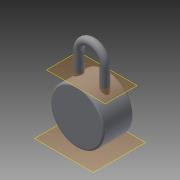
# Autodesk Inventor part: Noke
Saved by Autodesk Inventor 2015 SP2 (Build 190223200, 223)
## iProperties
Created: 2016-08-30
Part Number: Noke
Material: Generic
Document SubType Name: Modeling
Designer: jm799
Density: 1 g/cm^3
Appearance: Default
Author: jm799
Autodesk Inventor part; units mm, degrees
ref_plane "YZ Plane" through (0, 0, 0) normal (1, 0, 0) x (0, 1, 0)
ref_plane "XZ Plane" through (0, 0, 0) normal (0, 1, 0) x (-1, 0, 0)
sketch "Sketch1" plane through (0, 0, 0) normal (0, 1, 0) x (-1, 0, 0)
  circle A0 centre (0, 0) radius 27.375
  dimension "d0" = 54.75
  constraints: 1 centre point, 1 coincident
  measures "d0" diameter of A0
extrude "Extrusion1" add sketch "Sketch1" along normal blind 29.57
sketch "Sketch2" plane through (0, 29.57, 0) normal (0, 1, 0) x (1, 0, 0)
  point P0 (0, 0)
ref_plane "Work Plane1" through (0, 0, 27.375) normal (0, 0, 1) x (1, 0, 0)
sketch "Sketch3" plane through (0, 0, 27.375) normal (0, 0, 1) x (1, 0, 0)
  line L0 (-27.375, 0) -> (27.375, 0) construction
  line L1 (27.375, 0) -> (27.375, 29.57) construction
  line L2 (27.375, 0) -> (27.375, 29.57) construction
  line L3 (27.375, 29.57) -> (-27.375, 29.57) construction
  line L4 (-17.35, 14.785) -> (17.35, 14.785)
  circle A0 centre (13.3672, 14.785) radius 4
  line L5 (0, 0) -> (0, 29.57) construction
  circle A1 centre (-13.3672, 14.785) radius 4
  point P0 (0, 0)
  point P1 (0, 14.785)
  dimension "d3" = 34.7
  dimension "d4" = 8
  constraints: 7 end point, 3 midpoint, 2 centre point, 2 point on line, 1 horizontal, 1 perpendicular, 1 symmetric about line, 1 vertical alignment, 1 other
  measures "d3" distance of L4.start L4.end
  measures "d4" diameter of A0
extrude "Extrusion2" add sketch "Sketch3" against normal blind 10 and the other way blind 18
sketch "Sketch4" plane through (13.3672, 14.785, 45.375) normal (0, 0, 1) x (1, 0, 0)
  line L0 (-13.3672, -26.0897) -> (-13.3672, 22.3589)
  point P0 (-13.3672, -14.785)
  constraints: 2 end point, 1 vertical
sketch "Sketch5" plane through (13.3672, 14.785, 45.375) normal (0, 0, 1) x (1, 0, 0)
  circle A0 centre (0, 0) radius 4
  line L0 (-13.3672, 32.0486) -> (-13.3672, -35.7794) projected
  point P0 (-13.3672, -14.785)
  dimension "d9" = 8
  constraints: 1 centre point
  measures "d9" diameter of A0
revolve "Revolution1" add sketch "Sketch5" angle 180 about axis through (0, 37.1439, 45.375) along (0, -1, 0)
sketch "Sketch8" plane through (0, 0, 0) normal (0, -1, 0) x (1, 0, 0)
  circle A0 centre (0, 0) radius 26.75
  dimension "d11" = 53.5
  constraints: 1 centre point, 1 coincident
  measures "d11" diameter of A0
sketch "Sketch9" plane through (0, 29.57, 0) normal (0, 1, 0) x (1, 0, 0)
  circle A0 centre (0, 0) radius 26.75
  dimension "d12" = 53.5
  constraints: 1 centre point, 1 coincident
  measures "d12" diameter of A0
extrude "Extrusion3" add sketch "Sketch9" along normal blind 0.5
extrude "Extrusion4" add sketch "Sketch8" along normal blind 0.5
fillet "Fillet1" radius 2 1 edges at (-26.75, -0.5, 0)
fillet "Fillet2" radius 1.5 1 edges at (27.375, 0, 0)
fillet "Fillet3" radius 1.5 1 edges at (27.375, 29.57, 0)
fillet "Fillet4" radius 1 1 edges at (-26.75, 30.07, 0)
ref_plane "Work Plane2" through (0, 0, -27.375) normal (0, 0, 1) x (1, 0, 0)
sketch "Sketch10" plane through (0, 0, -27.375) normal (0, 0, 1) x (1, 0, 0)
  line L0 (27.375, 28.3517) -> (-27.375, 28.3517) construction
  line L1 (27.3423, 28.3517) -> (-27.3423, 28.3517) construction
  line L2 (27.375, 28.3517) -> (27.375, 1.2183) construction
  line L3 (-27.375, 1.2183) -> (27.375, 1.2183) construction
  line L4 (27.375, 1.2183) -> (27.375, 28.3517) construction
  circle A0 centre (0, 14.785) radius 7.5
  circle A1 centre (0, 14.785) radius 6.5
  line L5 (1.0367, 18.8545) -> (1.0367, 10.785)
  line L6 (-13.3672, 10.785) -> (13.3672, 10.785) projected
  line L7 (0, 28.3517) -> (0, 1.2183) construction
  line L8 (-1.0367, 18.8545) -> (-1.0367, 10.785)
  arc A2 (1.0367, 18.8545) -> (-1.0367, 18.8545) centre (0, 18.8545) ccw construction
  arc A3 (-1.0367, 10.785) -> (1.0367, 10.785) centre (0, 10.785) ccw construction
  arc A4 (1.0367, 18.8545) -> (-1.0367, 18.8545) centre (0, 18.8545) ccw
  arc A5 (-1.0367, 10.785) -> (1.0367, 10.785) centre (0, 10.785) ccw
  point P0 (0, 0)
  point P1 (0, 14.785)
  point P2 (27.375, 14.785)
  dimension "d21" = 15
  dimension "d22" = 13
  constraints: 11 end point, 8 point on circle, 6 centre point, 6 tangent, 4 midpoint, 3 point on line, 2 symmetric about line, 1 coincident, 1 collinear, 1 horizontal alignment, 1 vertical, 1 vertical alignment
  measures "d21" diameter of A0
  measures "d22" diameter of A1
extrude "Extrusion5" add sketch "Sketch10" against normal blind 0.5 contours L6 A5 A1 | A1 L6 L5 A4 L8
sketch "Sketch11" plane through (0, 0, -27.375) normal (0, 0, 1) x (1, 0, 0)
  circle A0 centre (0, 14.7302) radius 7.4566
  point P0 (0, 0)
  constraints: 1 centre point
extrude "Extrusion6" add sketch "Sketch11" along normal blind 1
body "Solid1"
